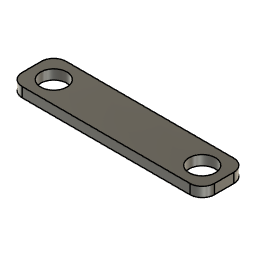
L1.1 (Autodesk Fusion 360 design; units mm, degrees)
Autodesk Fusion 360 part; units mm, degrees
sketch "Sketch1" plane through (0, 0, 0) normal (0, 0, 1) x (1, 0, 0)
  line L0 (19.75, 4.5) -> (-19.75, 4.5)
  line L1 (-19.75, 4.5) -> (-19.75, -4.5)
  line L2 (-19.75, -4.5) -> (19.75, -4.5)
  line L3 (19.75, -4.5) -> (19.75, 4.5)
  line L4 (19.75, 4.5) -> (-19.75, -4.5) construction
  line L5 (-19.75, 4.5) -> (19.75, -4.5) construction
  dimension "d1" = 39.5
  dimension "d2" = 9
  constraint horizontal L0
  constraint perpendicular L0 L1
  constraint parallel L0 L2
  constraint parallel L1 L3
  constraint coincident L4 origin
  constraint coincident L5 origin
  measures "d1" distance of L1.end L2.end
  measures "d2" distance of L0.end L1.end
extrude "Extrude1" add sketch "Sketch1" along normal blind 2
fillet "Fillet1" radius 2.5 4 edges at (-19.75, -4.5, 1) (-19.75, 4.5, 1) (19.75, 4.5, 1) (19.75, -4.5, 1)
sketch "Sketch2" plane through (0, 0, 2) normal (0, 0, 1) x (-1, 0, 0)
  arc A0 (-17.25, 4.5) -> (-19.75, 2) centre (-17.25, 2) ccw
  line L0 (-17.25, -4.5) -> (17.25, -4.5)
  arc A1 (17.25, -4.5) -> (19.75, -2) centre (17.25, -2) ccw
  line L1 (17.25, 4.5) -> (-17.25, 4.5)
  line L2 (-19.75, 2) -> (-19.75, -2)
  arc A2 (-19.75, -2) -> (-17.25, -4.5) centre (-17.25, -2) ccw
  line L3 (19.75, -2) -> (19.75, 2)
  arc A3 (19.75, 2) -> (17.25, 4.5) centre (17.25, 2) ccw
  line L4 (19.75, 0) -> (-19.75, 0) construction
  line L5 (19.75, 0) -> (15.25, 0)
  line L6 (-19.75, 0) -> (-15.25, 0)
  circle A4 centre (15.25, 0) radius 2.7
  circle A5 centre (-15.25, 0) radius 2.7
  dimension "d11" = 4.5
  dimension "d12" = 4.5
  dimension "d13" = 5.4
  dimension "d14" = 5.4
  constraint midpoint L3 L4.start
  constraint midpoint L2 L4.end
  constraint perpendicular L3 L5
  constraint perpendicular L2 L6
  constraint coincident L5.end A4.centre
  constraint coincident L6.end A5.centre
  measures "d11" distance of L4.start L5.end
  measures "d12" distance of L4.end L6.end
  measures "d13" diameter of A4
  measures "d14" diameter of A5
extrude "Extrude2" cut sketch "Sketch2" against normal blind 3 contours A4 | A5
